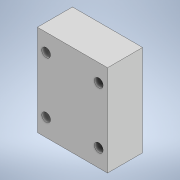
# Autodesk Inventor part: Soporte Linear Rail X
Saved by Autodesk Inventor 2021 (Build 250183000, 183)
## iProperties
Created: 2023-01-21
Part Number: Soporte Linear Rail X
Material: Genérico
Document SubType Name: Modeling
Designer: Diego.labarca
Density: 1 g/cm^3
Appearance: Valor por defecto
Author: Diego.labarca
Autodesk Inventor part; units mm, degrees
ref_plane "YZ Plane" through (0, 0, 0) normal (1, 0, 0) x (0, 1, 0)
ref_plane "XZ Plane" through (0, 0, 0) normal (0, 1, 0) x (-1, 0, 0)
ref_plane "XY Plane" through (0, 0, 0) normal (0, 0, 1) x (1, 0, 0)
sketch "Boceto1" plane through (0, 0, 0) normal (0, 0, 1) x (1, 0, 0)
  line L0 (-10, 13) -> (10, 13)
  line L1 (10, 13) -> (10, -13)
  line L2 (10, -13) -> (-10, -13)
  line L3 (-10, -13) -> (-10, 13)
  circle A0 centre (7.5, 8) radius 1.25
  circle A1 centre (-7.5, 8) radius 1.25
  circle A2 centre (7.5, -8) radius 1.25
  circle A3 centre (-7.5, -8) radius 1.25
  line L4 (1.6972, 0) -> (0, 0)
  line L5 (0, 0) -> (0, 1.3941)
  dimension "d0" = 2.5
  dimension "d3" = 15
  dimension "d6" = 16
  dimension "d9" = 7.5
  dimension "d10" = 8
  dimension "d11" = 26
  dimension "d12" = 20
  constraints: 12 end point, 4 centre point, 3 horizontal, 2 parallel, 2 perpendicular, 1 vertical, 8 other
  measures "d0" diameter of A0
  measures "d3" distance of A0.centre A1.centre
  measures "d6" distance of A0.centre A2.centre
  measures "d9" distance from line of A0.centre L5
  measures "d10" distance from line of L4 A2.centre
  measures "d11" distance of L0.end L1.end
  measures "d12" distance of L0.start L0.end
extrude "Extrusión1" add sketch "Boceto1" along normal blind 10
equation "\"d9\" = 0.5 * d3"
equation "\"d10\" = 0.5 * d6"
